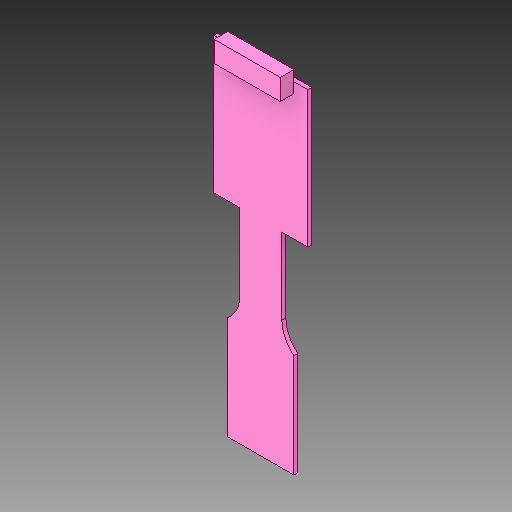
# Autodesk Inventor part: Circuit_center
Saved by Autodesk Inventor 2018 (Build 220112000, 112)
## iProperties
Created: 2018-05-04
Part Number: Circuit_center
Material: Generic
Document SubType Name: Modeling
Designer: suchanek
Density: 1 g/cm^3
Appearance: Default
Mass: 1.7923 g
Surface Area: 34.5913 cm^2
Volume: 1.7923 cm^3
Author: suchanek
Autodesk Inventor part; units mm, degrees
ref_plane "YZ Plane" through (0, 0, 0) normal (1, 0, 0) x (0, 1, 0)
ref_plane "XZ Plane" through (0, 0, 0) normal (0, 1, 0) x (-1, 0, 0)
ref_plane "XY Plane" through (0, 0, 0) normal (0, 0, 1) x (1, 0, 0)
sketch "Sketch1" plane through (0, 0, 0) normal (0, 0, 1) x (1, 0, 0)
  line L0 (0, 0) -> (23.5, 0)
  line L1 (23.5, 0) -> (23.5, 24.1419)
  line L2 (23.5, 85) -> (0, 85)
  line L3 (0, 85) -> (0, 51)
  line L4 (-1.5, 51) -> (0, 51)
  line L5 (6.5, 51) -> (6.5, 32)
  line L6 (-1.5, 24) -> (-1.5, 24)
  line L7 (-1.5, 24) -> (-1.5, 51)
  arc A0 (-1.5, 24) -> (0, 24.1419) centre (-1.5, 32) ccw
  line L8 (11.75, 79.5403) -> (11.75, 67.8807)
  line L9 (25, 51) -> (23.5, 51)
  line L10 (17, 51) -> (17, 32)
  line L11 (25, 24) -> (25, 24)
  line L12 (25, 24) -> (25, 51)
  arc A1 (17, 32) -> (20, 25.755) centre (25, 32) ccw
  line L13 (0, 51) -> (6.5, 51)
  line L14 (0, 51) -> (0, 24.1419)
  line L15 (0, 24.1419) -> (0, 0)
  arc A2 (0, 24.1419) -> (3.5, 25.755) centre (-1.5, 32) ccw
  line L16 (23.5, 24.1419) -> (23.5, 51)
  arc A3 (23.5, 24.1419) -> (25, 24) centre (25, 32) ccw
  line L17 (23.5, 51) -> (23.5, 85)
  line L18 (23.5, 51) -> (17, 51)
  line L19 (3.5, 25.755) -> (3.5, 0)
  arc A4 (3.5, 25.755) -> (6.5, 32) centre (-1.5, 32) ccw
  line L20 (20, 25.755) -> (20, 0)
  arc A5 (20, 25.755) -> (23.5, 24.1419) centre (25, 32) ccw
  dimension "d0" = 23.5
  dimension "d1" = 85
  dimension "d8" = 8
  dimension "d9" = 6.5
  dimension "d10" = 19
  dimension "d11" = 32
  dimension "d12" = 3.5
  constraints: 42 end point, 13 parallel, 12 point on circle, 7 perpendicular, 6 centre point, 6 symmetric about line, 4 horizontal, 4 tangent, 3 point on line, 1 horizontal alignment, 1 vertical, 2 other
  measures "d0" distance of L0.start L0.end
  measures "d1" distance of L2.end L0.start
  measures "d8" radius of A0
  measures "d9" distance between parallel lines of L5 L3
  measures "d10" distance from line of L4 A0.centre
  measures "d11" distance from line of L0 A0.centre
  measures "d12" distance between parallel lines of L15 L19
extrude "Extrusion1" add sketch "Sketch1" along normal blind 1 contours L19 A4 L5 L13 L3 L2 L17 L18 L10 A1 L20 L0
sketch "Sketch2" plane through (0, 0, 1) normal (0, 0, 1) x (1, 0, 0)
  line L0 (3.495, 82.4) -> (20.005, 82.4)
  line L1 (20.005, 82.4) -> (20.005, 87.6)
  line L2 (20.005, 87.6) -> (3.495, 87.6)
  line L3 (3.495, 87.6) -> (3.495, 82.4)
  line L4 (11.75, 82.8889) -> (11.75, 86.7771)
  line L5 (23.5, 85) -> (0, 85) projected
  line L6 (0, 85) -> (0, 89.9158)
  line L7 (23.5, 85) -> (23.5, 89.26)
  point P0 (0, 0)
  dimension "d4" = 2.6
  dimension "d5" = 16.51
  constraints: 14 end point, 3 vertical, 2 parallel, 1 horizontal, 1 perpendicular, 3 other
  measures "d4" distance between parallel lines of L2 L5
  measures "d5" distance of L1.end L2.end
extrude "Extrusion2" add sketch "Sketch2" along normal blind 3.4
body "Solid1"
